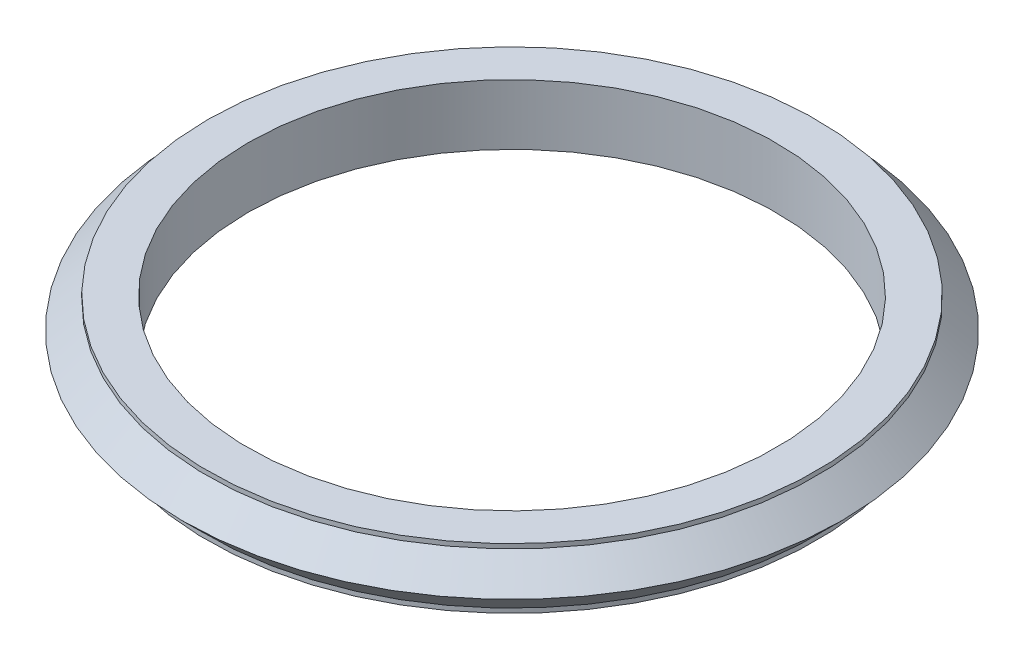
# Autodesk Inventor part: 3DPRINT,INNER-V
Saved by Autodesk Inventor 2026 (Build 300175000, 175)
## iProperties
Created: 2026-02-03
Part Number: 3DPRINT,INNER-V
Material: Nylon 6/6
Document SubType Name: Modeling
Designer: littl
Density: 1.13 g/cm^3
Appearance: Nylon 6
Author: littl
Autodesk Inventor part; units mm, degrees
ref_plane "YZ Plane" through (0, 0, 0) normal (1, 0, 0) x (0, 1, 0)
ref_plane "XZ Plane" through (0, 0, 0) normal (0, 1, 0) x (-1, 0, 0)
ref_plane "XY Plane" through (0, 0, 0) normal (0, 0, 1) x (1, 0, 0)
sketch "Sketch1" plane through (0, 0, 0) normal (0, 0, 1) x (1, 0, 0)
  line L0 (0, -8.2641) -> (0, 19.7359)
  line L1 (-162.5659, 0) -> (21.6343, 0) construction
  line L2 (-107.95, 8.89) -> (-107.95, -8.89) construction
  line L3 (-107.95, 8.89) -> (-90.3815, 8.89) construction
  line L4 (-90.3815, 8.89) -> (-90.3815, 7.3025) construction
  line L5 (-90.3815, 7.3025) -> (-91.504, 6.18) construction
  line L6 (-91.504, 6.18) -> (-92.9409, 7.6168) construction
  line L7 (-92.9409, 7.6168) -> (-95.186, 5.3717) construction
  line L8 (-95.186, 5.3717) -> (-93.7491, 3.9349) construction
  line L9 (-93.7491, 3.9349) -> (-97.684, 0) construction
  line L10 (-97.176, 0) -> (-84.8354, 12.3406) construction
  line L11 (-94.0634, 6.4943) -> (-92.3726, 4.8034) construction
  circle A0 centre (-93.218, 5.6489) radius 1.3081 construction
  line L12 (-90.3815, -8.89) -> (-90.3815, -7.3025) construction
  line L13 (-90.3815, -7.3025) -> (-91.504, -6.18) construction
  line L14 (-91.504, -6.18) -> (-92.9409, -7.6168) construction
  line L15 (-92.9409, -7.6168) -> (-95.186, -5.3717) construction
  line L16 (-95.186, -5.3717) -> (-93.7491, -3.9349) construction
  line L17 (-93.7491, -3.9349) -> (-97.684, 0) construction
  line L18 (-107.95, -8.89) -> (-90.3815, -8.89) construction
  line L19 (-89.6195, 8.89) -> (-89.6195, 7.5565)
  line L20 (-89.6195, 7.5565) -> (-97.176, 0)
  line L21 (-89.6195, 8.89) -> (-77.7875, 8.89)
  line L22 (-77.7875, 8.89) -> (-77.7875, -8.89)
  line L23 (-89.6195, -8.89) -> (-89.6195, -7.5565)
  line L24 (-89.6195, -7.5565) -> (-97.176, 0)
  line L25 (-89.6195, -8.89) -> (-77.7875, -8.89)
  point P0 (0, 0)
  point P1 (0, 0)
  point P2 (0, 0)
  dimension "d23" = 1.5875
  dimension "d24" = 2.032
  dimension "d25" = 45
  dimension "d26" = 0.508
  dimension "d27" = 3.175
  dimension "d28" = 2.6162
  dimension "d29" = 186.436
  dimension "d30" = 215.9
  dimension "d31" = 17.78
  dimension "d32" = 1.5875
  dimension "d33" = 0.762
  dimension "d34" = 155.575
  dimension "d35" = 17.78
  constraints: 52 end point, 10 symmetric about line, 9 point on line, 5 perpendicular, 3 vertical, 2 coincident, 2 horizontal, 2 midpoint, 1 centre point, 1 horizontal alignment, 1 parallel
  measures "d23" distance of L3.end L4.end
  measures "d24" distance of L5.end L6.end
  measures "d25" angle of L1 L9
  measures "d26" distance of L10.start L9.end
  measures "d27" distance of L6.end L7.end
  measures "d28" diameter of A0
  measures "d29" diameter of A0.centre L0
  measures "d30" diameter of L2 L0
  measures "d31" distance of L2.start L2.end
  measures "d32" distance of L4.end L5.end
  measures "d33" distance between parallel lines of L4 L19
  measures "d34" diameter of L22 L0
  measures "d35" distance of L21.end L22.end
revolve "Revolution1" add sketch "Sketch1" angle 360 about axis through (0, -8.2641, 0) along (0, 1, 0)
body "Solid1"
